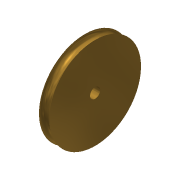
# Autodesk Inventor part: spool
Saved by Autodesk Inventor 2015 (Build 190159000, 159)
## iProperties
Created: 2015-01-22
Part Number: spool
Material: Generic
Document SubType Name: Modeling
Designer: rihoobler
Density: 1 g/cm^3
Appearance: Brass - Satin
Author: rihoobler
Autodesk Inventor part; units mm, degrees
ref_plane "YZ Plane" through (0, 0, 0) normal (1, 0, 0) x (0, 1, 0)
ref_plane "XZ Plane" through (0, 0, 0) normal (0, 1, 0) x (-1, 0, 0)
ref_plane "XY Plane" through (0, 0, 0) normal (0, 0, 1) x (1, 0, 0)
sketch "Sketch1" plane through (0, 0, 0) normal (0, 0, 1) x (1, 0, 0)
  line L0 (0, 0) -> (15.6296, 0)
  line L1 (3.7037, 1.5875) -> (6.8787, 1.5875)
  line L2 (6.8787, 1.5875) -> (6.8787, 14.2875)
  line L3 (3.7037, 14.2875) -> (3.7037, 1.5875)
  arc A0 (3.7037, 14.2875) -> (6.8787, 14.2875) centre (5.2912, 14.2875) ccw
  dimension "d0" = 3.175
  dimension "d1" = 12.7
  dimension "d2" = 1.5875
  constraints: 8 end point, 2 horizontal, 2 point on circle, 1 centre point, 1 parallel, 1 perpendicular
  measures "d0" distance of L3.start L2.end
  measures "d1" distance of L2.end L1.end
  measures "d2" distance between parallel lines of L0 L1
revolve "Revolution1" add sketch "Sketch1" angle 360 about axis through (0, 0, 0) along (1, 0, 0)
body "Solid1"
